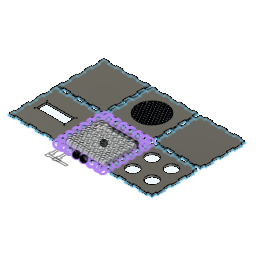
Alarm Clock v4 (Autodesk Fusion 360 design; units mm, degrees)
Autodesk Fusion 360 part; units mm, degrees
(part 1 of 3)
sketch "box (5)" plane through (0, 0, 0) normal (0, 0, 1) x (1, 0, 0)
  line L0 (0, 72.1875) -> (3, 72.1875)
  line L1 (0, 17.0625) -> (0, 3)
  line L2 (3, 108.9375) -> (3, 90.5625)
  line L3 (3, 35.4375) -> (3, 17.0625)
  line L4 (0, 108.9375) -> (3, 108.9375)
  line L5 (3, 72.1875) -> (3, 53.8125)
  line L6 (3, 53.8125) -> (0, 53.8125)
  line L7 (0, 35.4375) -> (3, 35.4375)
  line L8 (3, 17.0625) -> (0, 17.0625)
  line L9 (3, 90.5625) -> (0, 90.5625)
  line L10 (0, 123) -> (0, 108.9375)
  line L11 (0, 53.8125) -> (0, 35.4375)
  line L12 (117, 35.4375) -> (120, 35.4375)
  line L13 (120, 123) -> (105.9375, 123)
  line L14 (32.4375, 3) -> (50.8125, 3)
  line L15 (50.8125, 6) -> (69.1875, 6)
  line L16 (69.1875, 6) -> (69.1875, 3)
  line L17 (120, 108.9375) -> (120, 123)
  line L18 (87.5625, 3) -> (87.5625, 6)
  line L19 (120, 3) -> (120, 17.0625)
  line L20 (120, 53.8125) -> (117, 53.8125)
  line L21 (117, 53.8125) -> (117, 72.1875)
  line L22 (0, 90.5625) -> (0, 72.1875)
  line L23 (69.1875, 3) -> (87.5625, 3)
  line L24 (120, 90.5625) -> (117, 90.5625)
  line L25 (0, 3) -> (14.0625, 3)
  line L26 (87.5625, 123) -> (69.1875, 123)
  line L27 (50.8125, 3) -> (50.8125, 6)
  line L28 (87.5625, 120) -> (87.5625, 123)
  line L29 (87.5625, 6) -> (105.9375, 6)
  line L30 (105.9375, 6) -> (105.9375, 3)
  line L31 (120, 35.4375) -> (120, 53.8125)
  line L32 (120, 17.0625) -> (117, 17.0625)
  line L33 (120, 72.1875) -> (120, 90.5625)
  line L34 (105.9375, 120) -> (87.5625, 120)
  line L35 (32.4375, 6) -> (32.4375, 3)
  line L36 (14.0625, 3) -> (14.0625, 6)
  line L37 (117, 17.0625) -> (117, 35.4375)
  line L38 (117, 90.5625) -> (117, 108.9375)
  line L39 (105.9375, 123) -> (105.9375, 120)
  line L40 (14.0625, 6) -> (32.4375, 6)
  line L41 (105.9375, 3) -> (120, 3)
  line L42 (117, 72.1875) -> (120, 72.1875)
  line L43 (117, 108.9375) -> (120, 108.9375)
  line L44 (69.1875, 123) -> (69.1875, 120)
  line L45 (14.0625, 123) -> (0, 123)
  line L46 (14.0625, 120) -> (14.0625, 123)
  line L47 (32.4375, 123) -> (32.4375, 120)
  line L48 (32.4375, 120) -> (14.0625, 120)
  line L49 (50.8125, 123) -> (32.4375, 123)
  line L50 (50.8125, 120) -> (50.8125, 123)
  line L51 (69.1875, 120) -> (50.8125, 120)
  line L52 (210.5625, 123) -> (192.1875, 123)
  line L53 (173.8125, 3) -> (173.8125, 6)
  line L54 (240, 123) -> (228.9375, 123)
  line L55 (210.5625, 3) -> (210.5625, 6)
  line L56 (243, 35.4375) -> (240, 35.4375)
  line L57 (123, 90.5625) -> (126, 90.5625)
  line L58 (210.5625, 6) -> (228.9375, 6)
  line L59 (126, 3) -> (137.0625, 3)
  line L60 (192.1875, 123) -> (192.1875, 120)
  line L61 (123, 35.4375) -> (123, 17.0625)
  line L62 (123, 17.0625) -> (126, 17.0625)
  line L63 (126, 108.9375) -> (123, 108.9375)
  line L64 (126, 90.5625) -> (126, 72.1875)
  line L65 (240, 108.9375) -> (240, 123)
  line L66 (243, 72.1875) -> (240, 72.1875)
  line L67 (155.4375, 6) -> (155.4375, 3)
  line L68 (173.8125, 120) -> (173.8125, 123)
  line L69 (123, 72.1875) -> (123, 53.8125)
  line L70 (240, 3) -> (240, 17.0625)
  line L71 (126, 53.8125) -> (126, 35.4375)
  line L72 (126, 17.0625) -> (126, 3)
  line L73 (243, 17.0625) -> (243, 35.4375)
  line L74 (228.9375, 6) -> (228.9375, 3)
  line L75 (123, 108.9375) -> (123, 90.5625)
  line L76 (192.1875, 6) -> (192.1875, 3)
  line L77 (155.4375, 3) -> (173.8125, 3)
  line L78 (137.0625, 6) -> (155.4375, 6)
  line L79 (173.8125, 6) -> (192.1875, 6)
  line L80 (228.9375, 120) -> (210.5625, 120)
  line L81 (126, 123) -> (126, 108.9375)
  line L82 (137.0625, 3) -> (137.0625, 6)
  line L83 (126, 35.4375) -> (123, 35.4375)
  line L84 (126, 72.1875) -> (123, 72.1875)
  line L85 (123, 53.8125) -> (126, 53.8125)
  line L86 (240, 17.0625) -> (243, 17.0625)
  line L87 (240, 35.4375) -> (240, 53.8125)
  line L88 (243, 108.9375) -> (240, 108.9375)
  line L89 (173.8125, 123) -> (155.4375, 123)
  line L90 (240, 53.8125) -> (243, 53.8125)
  line L91 (192.1875, 120) -> (173.8125, 120)
  line L92 (243, 53.8125) -> (243, 72.1875)
  line L93 (240, 90.5625) -> (243, 90.5625)
  line L94 (240, 72.1875) -> (240, 90.5625)
  line L95 (137.0625, 123) -> (126, 123)
  line L96 (155.4375, 120) -> (137.0625, 120)
  line L97 (210.5625, 120) -> (210.5625, 123)
  line L98 (243, 90.5625) -> (243, 108.9375)
  line L99 (155.4375, 123) -> (155.4375, 120)
  line L100 (228.9375, 3) -> (240, 3)
  line L101 (137.0625, 120) -> (137.0625, 123)
  line L102 (228.9375, 123) -> (228.9375, 120)
  line L103 (192.1875, 3) -> (210.5625, 3)
  line L104 (249, 120) -> (249, 108.9375)
  line L105 (260.0625, 6) -> (260.0625, 3)
  line L106 (351.9375, 3) -> (351.9375, 6)
  line L107 (296.8125, 6) -> (296.8125, 3)
  line L108 (278.4375, 6) -> (296.8125, 6)
  line L109 (366, 72.1875) -> (363, 72.1875)
  line L110 (363, 108.9375) -> (363, 120)
  line L111 (333.5625, 6) -> (333.5625, 3)
  line L112 (249, 17.0625) -> (249, 6)
  line L113 (278.4375, 3) -> (278.4375, 6)
  line L114 (351.9375, 6) -> (363, 6)
  line L115 (333.5625, 120) -> (315.1875, 120)
  line L116 (366, 108.9375) -> (363, 108.9375)
  line L117 (246, 72.1875) -> (246, 53.8125)
  line L118 (351.9375, 120) -> (351.9375, 123)
  line L119 (246, 17.0625) -> (249, 17.0625)
  line L120 (315.1875, 120) -> (315.1875, 123)
  line L121 (296.8125, 123) -> (296.8125, 120)
  line L122 (260.0625, 120) -> (249, 120)
  line L123 (366, 90.5625) -> (366, 108.9375)
  line L124 (249, 90.5625) -> (249, 72.1875)
  line L125 (246, 108.9375) -> (246, 90.5625)
  line L126 (366, 35.4375) -> (363, 35.4375)
  line L127 (246, 90.5625) -> (249, 90.5625)
  line L128 (363, 35.4375) -> (363, 53.8125)
  line L129 (296.8125, 3) -> (315.1875, 3)
  line L130 (278.4375, 123) -> (260.0625, 123)
  line L131 (249, 6) -> (260.0625, 6)
  line L132 (315.1875, 6) -> (333.5625, 6)
  line L133 (246, 53.8125) -> (249, 53.8125)
  line L134 (260.0625, 3) -> (278.4375, 3)
  line L135 (363, 120) -> (351.9375, 120)
  line L136 (363, 6) -> (363, 17.0625)
  line L137 (333.5625, 123) -> (333.5625, 120)
  line L138 (249, 108.9375) -> (246, 108.9375)
  line L139 (363, 90.5625) -> (366, 90.5625)
  line L140 (315.1875, 123) -> (296.8125, 123)
  line L141 (363, 72.1875) -> (363, 90.5625)
  line L142 (366, 53.8125) -> (366, 72.1875)
  line L143 (315.1875, 3) -> (315.1875, 6)
  line L144 (296.8125, 120) -> (278.4375, 120)
  line L145 (249, 53.8125) -> (249, 35.4375)
  line L146 (260.0625, 123) -> (260.0625, 120)
  line L147 (278.4375, 120) -> (278.4375, 123)
  line L148 (249, 35.4375) -> (246, 35.4375)
  line L149 (246, 35.4375) -> (246, 17.0625)
  line L150 (249, 72.1875) -> (246, 72.1875)
  line L151 (333.5625, 3) -> (351.9375, 3)
  line L152 (351.9375, 123) -> (333.5625, 123)
  line L153 (363, 17.0625) -> (366, 17.0625)
  line L154 (363, 53.8125) -> (366, 53.8125)
  line L155 (366, 17.0625) -> (366, 35.4375)
  line L156 (3, 213.5625) -> (0, 213.5625)
  line L157 (0, 231.9375) -> (3, 231.9375)
  line L158 (3, 231.9375) -> (3, 213.5625)
  line L159 (0, 195.1875) -> (3, 195.1875)
  line L160 (32.4375, 243) -> (14.0625, 243)
  line L161 (14.0625, 129) -> (32.4375, 129)
  line L162 (0, 140.0625) -> (0, 126)
  line L163 (69.1875, 126) -> (87.5625, 126)
  line L164 (50.8125, 126) -> (50.8125, 129)
  line L165 (69.1875, 129) -> (69.1875, 126)
  line L166 (120, 176.8125) -> (117, 176.8125)
  line L167 (117, 140.0625) -> (117, 158.4375)
  line L168 (0, 176.8125) -> (0, 158.4375)
  line L169 (14.0625, 246) -> (0, 246)
  line L170 (87.5625, 126) -> (87.5625, 129)
  line L171 (3, 195.1875) -> (3, 176.8125)
  line L172 (50.8125, 243) -> (50.8125, 246)
  line L173 (0, 213.5625) -> (0, 195.1875)
  line L174 (69.1875, 243) -> (50.8125, 243)
  line L175 (120, 246) -> (105.9375, 246)
  line L176 (117, 231.9375) -> (120, 231.9375)
  line L177 (120, 158.4375) -> (120, 176.8125)
  line L178 (87.5625, 129) -> (105.9375, 129)
  line L179 (32.4375, 126) -> (50.8125, 126)
  line L180 (0, 126) -> (14.0625, 126)
  line L181 (32.4375, 129) -> (32.4375, 126)
  line L182 (105.9375, 246) -> (105.9375, 243)
  line L183 (105.9375, 243) -> (87.5625, 243)
  line L184 (120, 140.0625) -> (117, 140.0625)
  line L185 (87.5625, 243) -> (87.5625, 246)
  line L186 (87.5625, 246) -> (69.1875, 246)
  line L187 (3, 158.4375) -> (3, 140.0625)
  line L188 (120, 195.1875) -> (120, 213.5625)
  line L189 (117, 213.5625) -> (117, 231.9375)
  line L190 (117, 195.1875) -> (120, 195.1875)
  line L191 (69.1875, 246) -> (69.1875, 243)
  line L192 (32.4375, 246) -> (32.4375, 243)
  line L193 (0, 158.4375) -> (3, 158.4375)
  line L194 (50.8125, 129) -> (69.1875, 129)
  line L195 (14.0625, 126) -> (14.0625, 129)
  line L196 (120, 126) -> (120, 140.0625)
  line L197 (120, 213.5625) -> (117, 213.5625)
  line L198 (3, 140.0625) -> (0, 140.0625)
  line L199 (105.9375, 129) -> (105.9375, 126)
  line L200 (3, 176.8125) -> (0, 176.8125)
  line L201 (117, 176.8125) -> (117, 195.1875)
  line L202 (0, 246) -> (0, 231.9375)
  line L203 (14.0625, 243) -> (14.0625, 246)
  line L204 (50.8125, 246) -> (32.4375, 246)
  line L205 (120, 231.9375) -> (120, 246)
  line L206 (117, 158.4375) -> (120, 158.4375)
  line L207 (105.9375, 126) -> (120, 126)
  line L208 (126, 140.0625) -> (126, 126)
  line L209 (123, 140.0625) -> (126, 140.0625)
  line L210 (123, 158.4375) -> (123, 140.0625)
  line L211 (126, 158.4375) -> (123, 158.4375)
  line L212 (126, 195.1875) -> (123, 195.1875)
  line L213 (123, 213.5625) -> (126, 213.5625)
  line L214 (126, 231.9375) -> (123, 231.9375)
  line L215 (123, 176.8125) -> (126, 176.8125)
  line L216 (126, 176.8125) -> (126, 158.4375)
  line L217 (123, 195.1875) -> (123, 176.8125)
  line L218 (126, 213.5625) -> (126, 195.1875)
  line L219 (126, 246) -> (126, 231.9375)
  line L220 (137.0625, 126) -> (137.0625, 129)
  line L221 (173.8125, 126) -> (173.8125, 129)
  line L222 (192.1875, 129) -> (192.1875, 126)
  line L223 (137.0625, 129) -> (155.4375, 129)
  line L224 (155.4375, 126) -> (173.8125, 126)
  line L225 (123, 231.9375) -> (123, 213.5625)
  line L226 (240, 213.5625) -> (243, 213.5625)
  line L227 (240, 246) -> (228.9375, 246)
  line L228 (240, 158.4375) -> (240, 176.8125)
  line L229 (192.1875, 246) -> (192.1875, 243)
  line L230 (126, 126) -> (137.0625, 126)
  line L231 (243, 195.1875) -> (240, 195.1875)
  line L232 (228.9375, 129) -> (228.9375, 126)
  line L233 (243, 176.8125) -> (243, 195.1875)
  line L234 (137.0625, 246) -> (126, 246)
  line L235 (228.9375, 126) -> (240, 126)
  line L236 (210.5625, 126) -> (210.5625, 129)
  line L237 (240, 195.1875) -> (240, 213.5625)
  line L238 (228.9375, 246) -> (228.9375, 243)
  line L239 (243, 213.5625) -> (243, 231.9375)
  line L240 (155.4375, 246) -> (155.4375, 243)
  line L241 (240, 231.9375) -> (240, 246)
  line L242 (228.9375, 243) -> (210.5625, 243)
  line L243 (240, 126) -> (240, 140.0625)
  line L244 (243, 158.4375) -> (240, 158.4375)
  line L245 (243, 231.9375) -> (240, 231.9375)
  line L246 (155.4375, 243) -> (137.0625, 243)
  line L247 (210.5625, 129) -> (228.9375, 129)
  line L248 (240, 140.0625) -> (243, 140.0625)
  line L249 (137.0625, 243) -> (137.0625, 246)
  line L250 (192.1875, 243) -> (173.8125, 243)
  line L251 (155.4375, 129) -> (155.4375, 126)
  line L252 (192.1875, 126) -> (210.5625, 126)
  line L253 (173.8125, 129) -> (192.1875, 129)
  line L254 (243, 140.0625) -> (243, 158.4375)
  line L255 (210.5625, 246) -> (192.1875, 246)
  line L256 (210.5625, 243) -> (210.5625, 246)
  line L257 (240, 176.8125) -> (243, 176.8125)
  line L258 (173.8125, 246) -> (155.4375, 246)
  line L259 (173.8125, 243) -> (173.8125, 246)
  line L260 (296.8125, 129) -> (296.8125, 126)
  line L261 (260.0625, 126) -> (278.4375, 126)
  line L262 (278.4375, 126) -> (278.4375, 129)
  line L263 (249, 176.8125) -> (249, 158.4375)
  line L264 (249, 195.1875) -> (246, 195.1875)
  line L265 (296.8125, 126) -> (315.1875, 126)
  line L266 (249, 140.0625) -> (249, 129)
  line L267 (246, 231.9375) -> (246, 213.5625)
  line L268 (249, 129) -> (260.0625, 129)
  line L269 (246, 140.0625) -> (249, 140.0625)
  line L270 (246, 195.1875) -> (246, 176.8125)
  line L271 (278.4375, 129) -> (296.8125, 129)
  line L272 (315.1875, 126) -> (315.1875, 129)
  line L273 (260.0625, 129) -> (260.0625, 126)
  line L274 (315.1875, 129) -> (333.5625, 129)
  line L275 (333.5625, 129) -> (333.5625, 126)
  line L276 (246, 158.4375) -> (246, 140.0625)
  line L277 (249, 213.5625) -> (249, 195.1875)
  line L278 (351.9375, 246) -> (333.5625, 246)
  line L279 (249, 231.9375) -> (246, 231.9375)
  line L280 (333.5625, 126) -> (351.9375, 126)
  line L281 (249, 243) -> (249, 231.9375)
  line L282 (246, 213.5625) -> (249, 213.5625)
  line L283 (351.9375, 126) -> (351.9375, 129)
  line L284 (246, 176.8125) -> (249, 176.8125)
  line L285 (249, 158.4375) -> (246, 158.4375)
  line L286 (363, 176.8125) -> (366, 176.8125)
  line L287 (296.8125, 243) -> (278.4375, 243)
  line L288 (351.9375, 129) -> (363, 129)
  line L289 (278.4375, 246) -> (260.0625, 246)
  line L290 (296.8125, 246) -> (296.8125, 243)
  line L291 (363, 243) -> (351.9375, 243)
  line L292 (278.4375, 243) -> (278.4375, 246)
  line L293 (315.1875, 243) -> (315.1875, 246)
  line L294 (366, 140.0625) -> (366, 158.4375)
  line L295 (363, 158.4375) -> (363, 176.8125)
  line L296 (363, 231.9375) -> (363, 243)
  line L297 (366, 158.4375) -> (363, 158.4375)
  line L298 (363, 213.5625) -> (366, 213.5625)
  line L299 (366, 176.8125) -> (366, 195.1875)
  line L300 (363, 195.1875) -> (363, 213.5625)
  line L301 (315.1875, 246) -> (296.8125, 246)
  line L302 (351.9375, 243) -> (351.9375, 246)
  line L303 (363, 129) -> (363, 140.0625)
  line L304 (366, 231.9375) -> (363, 231.9375)
  line L305 (366, 195.1875) -> (363, 195.1875)
  line L306 (333.5625, 246) -> (333.5625, 243)
  line L307 (260.0625, 246) -> (260.0625, 243)
  line L308 (260.0625, 243) -> (249, 243)
  line L309 (363, 140.0625) -> (366, 140.0625)
  line L310 (366, 213.5625) -> (366, 231.9375)
  line L311 (333.5625, 243) -> (315.1875, 243)
sketch "Sketch2" plane through (0, 0, 0) normal (0, 0, 1) x (1, 0, 0)
  line L0 (246, 108.9375) -> (246, 90.5625)
  line L1 (249, 108.9375) -> (246, 108.9375)
  line L2 (249, 120) -> (249, 108.9375)
  line L3 (260.0625, 120) -> (249, 120)
  line L4 (278.4375, 123) -> (260.0625, 123)
  line L5 (260.0625, 123) -> (260.0625, 120)
  line L6 (278.4375, 120) -> (278.4375, 123)
  line L7 (351.9375, 123) -> (333.5625, 123)
  line L8 (363, 120) -> (351.9375, 120)
  line L9 (366, 90.5625) -> (366, 108.9375)
  line L10 (363, 108.9375) -> (363, 120)
  line L11 (366, 108.9375) -> (363, 108.9375)
  line L12 (351.9375, 120) -> (351.9375, 123)
  line L13 (249, 17.0625) -> (249, 6)
  line L14 (246, 17.0625) -> (249, 17.0625)
  line L15 (246, 35.4375) -> (246, 17.0625)
  line L16 (249, 6) -> (260.0625, 6)
  line L17 (260.0625, 6) -> (260.0625, 3)
  line L18 (260.0625, 3) -> (278.4375, 3)
  line L19 (333.5625, 3) -> (351.9375, 3)
  line L20 (351.9375, 3) -> (351.9375, 6)
  line L21 (351.9375, 6) -> (363, 6)
  line L22 (363, 6) -> (363, 17.0625)
  line L23 (363, 17.0625) -> (366, 17.0625)
  line L24 (366, 17.0625) -> (366, 35.4375)
  line L25 (260.0625, 123) -> (240, 123)
  line L26 (246, 108.9375) -> (246, 123)
  line L27 (351.9375, 123) -> (370, 123)
  line L28 (366, 108.9375) -> (366, 123)
  line L29 (246, 17.0625) -> (246, 0)
  line L30 (260.0625, 3) -> (246, 3)
  line L31 (351.9375, 3) -> (370, 3)
  line L32 (366, 17.0625) -> (366, 3)
  circle A0 centre (281.3553, 38.3553) radius 15
  line L33 (281.3553, 38.3553) -> (246, 3) construction
  circle A1 centre (330.6447, 38.3553) radius 15
  line L34 (330.6447, 38.3553) -> (366, 3) construction
  circle A2 centre (330.6447, 87.6447) radius 15
  line L35 (366, 123) -> (330.6447, 87.6447) construction
  circle A3 centre (281.3553, 87.6447) radius 15
  line L36 (246, 123) -> (281.3553, 87.6447) construction
  line L37 (246, 90.5625) -> (249, 90.5625)
  line L38 (249, 90.5625) -> (249, 72.1875)
  line L39 (249, 72.1875) -> (246, 72.1875)
  line L40 (246, 72.1875) -> (246, 53.8125)
  line L41 (246, 53.8125) -> (249, 53.8125)
  line L42 (249, 53.8125) -> (249, 35.4375)
  line L43 (249, 35.4375) -> (246, 35.4375)
  line L44 (296.8125, 120) -> (278.4375, 120)
  line L45 (315.1875, 123) -> (296.8125, 123)
  line L46 (296.8125, 123) -> (296.8125, 120)
  line L47 (315.1875, 120) -> (315.1875, 123)
  line L48 (333.5625, 120) -> (315.1875, 120)
  line L49 (333.5625, 123) -> (333.5625, 120)
  line L50 (363, 90.5625) -> (366, 90.5625)
  line L51 (363, 72.1875) -> (363, 90.5625)
  line L52 (366, 72.1875) -> (363, 72.1875)
  line L53 (366, 53.8125) -> (366, 72.1875)
  line L54 (363, 35.4375) -> (363, 53.8125)
  line L55 (363, 53.8125) -> (366, 53.8125)
  line L56 (366, 35.4375) -> (363, 35.4375)
  line L57 (333.5625, 6) -> (333.5625, 3)
  line L58 (315.1875, 6) -> (333.5625, 6)
  line L59 (315.1875, 3) -> (315.1875, 6)
  line L60 (296.8125, 3) -> (315.1875, 3)
  line L61 (296.8125, 6) -> (296.8125, 3)
  line L62 (278.4375, 6) -> (296.8125, 6)
  line L63 (278.4375, 3) -> (278.4375, 6)
  point P0 (249, 120)
  point P1 (249, 108.9375)
  point P2 (246, 108.9375)
  point P3 (246, 90.5625)
  point P4 (249, 90.5625)
  point P5 (249, 72.1875)
  point P6 (246, 72.1875)
  point P7 (246, 53.8125)
  point P8 (249, 53.8125)
  point P9 (249, 35.4375)
  point P10 (246, 35.4375)
  point P11 (246, 17.0625)
  point P12 (249, 17.0625)
  point P13 (249, 6)
  point P14 (260.0625, 6)
  point P15 (260.0625, 3)
  point P16 (278.4375, 3)
  point P17 (278.4375, 6)
  point P18 (296.8125, 6)
  point P19 (296.8125, 3)
  point P20 (315.1875, 3)
  point P21 (315.1875, 6)
  point P22 (333.5625, 6)
  point P23 (333.5625, 3)
  point P24 (351.9375, 3)
  point P25 (351.9375, 6)
  point P26 (363, 6)
  point P27 (363, 17.0625)
  point P28 (366, 17.0625)
  point P29 (366, 35.4375)
  point P30 (363, 35.4375)
  point P31 (363, 53.8125)
  point P32 (366, 53.8125)
  point P33 (366, 72.1875)
  point P34 (363, 72.1875)
  point P35 (363, 90.5625)
  point P36 (366, 90.5625)
  point P37 (366, 108.9375)
  point P38 (363, 108.9375)
  point P39 (363, 120)
  point P40 (351.9375, 120)
  point P41 (351.9375, 123)
  point P42 (333.5625, 123)
  point P43 (333.5625, 120)
  point P44 (315.1875, 120)
  point P45 (315.1875, 123)
  point P46 (296.8125, 123)
  point P47 (296.8125, 120)
  point P48 (278.4375, 120)
  point P49 (278.4375, 123)
  point P50 (260.0625, 123)
  point P51 (260.0625, 120)
  dimension "d1" = 30
  dimension "d2" = 50
  dimension "d3" = 45
  dimension "d4" = 30
  dimension "d5" = 50
  dimension "d6" = 45
  dimension "d7" = 30
  dimension "d8" = 50
  dimension "d9" = 45
  dimension "d10" = 30
  dimension "d11" = 50
  dimension "d12" = 45
  constraint coincident P50 L4.end
  constraint perpendicular L5 L25
  constraint coincident P2 L0.start
  constraint coincident L25 L26.end
  constraint perpendicular L25 L26
  constraint coincident P41 L7.start
  constraint perpendicular L12 L27
  constraint coincident P37 L9.end
  constraint coincident L27 L28.end
  constraint perpendicular L27 L28
  constraint coincident P11 L14.start
  constraint perpendicular L14 L29
  constraint coincident P15 L17.end
  constraint coincident L29 L30.end
  constraint perpendicular L29 L30
  constraint coincident P24 L19.end
  constraint perpendicular L20 L31
  constraint coincident P28 L23.end
  constraint coincident L31 L32.end
  constraint perpendicular L31 L32
  constraint coincident A0.centre L33.start
  constraint coincident A1.centre L34.start
  constraint coincident A2.centre L35.end
  constraint coincident A3.centre L36.end
  measures "d1" diameter of A0
  measures "d2" distance of L30.end A0.centre
  measures "d3" angle of L30 L33
  measures "d4" diameter of A1
  measures "d5" distance of L32.end A1.centre
  measures "d6" angle of L31 L34
  measures "d7" diameter of A2
  measures "d8" distance of L28.end A2.centre
  measures "d9" angle of L27 L35
  measures "d10" diameter of A3
  measures "d11" distance of L26.end A3.centre
  measures "d12" angle of L25 L36
extrude "Extrude1" add sketch "Sketch2" along normal blind 5.2 contours L0 L1 L2 L3 L4 L5 L6 L7 L8 L9 L10 L11 L12 L13 L14 L15 L16 L17 L18 L19 L20 L21 L22 L23 L24 L37 L38 L39 L40 L41 L42 L43 L44 L45 L46 L47 L48 L49 L50 L51 L52 L53 L54 L55 L56 L57 L58 L59 L60 L61 L62 L63 makes body 1
sketch "Sketch3" plane through (0, 0, 0) normal (0, 0, 1) x (1, 0, 0)
  line L0 (0, 123) -> (0, 108.9375)
  line L1 (14.0625, 123) -> (0, 123)
  line L2 (14.0625, 120) -> (14.0625, 123)
  line L3 (32.4375, 120) -> (14.0625, 120)
  line L4 (32.4375, 123) -> (32.4375, 120)
  line L5 (50.8125, 123) -> (32.4375, 123)
  line L6 (50.8125, 120) -> (50.8125, 123)
  line L7 (69.1875, 120) -> (50.8125, 120)
  line L8 (69.1875, 123) -> (69.1875, 120)
  line L9 (87.5625, 123) -> (69.1875, 123)
  line L10 (87.5625, 120) -> (87.5625, 123)
  line L11 (105.9375, 120) -> (87.5625, 120)
  line L12 (105.9375, 123) -> (105.9375, 120)
  line L13 (120, 123) -> (105.9375, 123)
  line L14 (120, 108.9375) -> (120, 123)
  line L15 (117, 108.9375) -> (120, 108.9375)
  line L16 (117, 90.5625) -> (117, 108.9375)
  line L17 (120, 90.5625) -> (117, 90.5625)
  line L18 (120, 72.1875) -> (120, 90.5625)
  line L19 (117, 53.8125) -> (117, 72.1875)
  line L20 (117, 72.1875) -> (120, 72.1875)
  line L21 (120, 53.8125) -> (117, 53.8125)
  line L22 (120, 35.4375) -> (120, 53.8125)
  line L23 (117, 35.4375) -> (120, 35.4375)
  line L24 (117, 17.0625) -> (117, 35.4375)
  line L25 (120, 17.0625) -> (117, 17.0625)
  line L26 (105.9375, 6) -> (105.9375, 3)
  line L27 (120, 3) -> (120, 17.0625)
  line L28 (105.9375, 3) -> (120, 3)
  line L29 (87.5625, 6) -> (105.9375, 6)
  line L30 (87.5625, 3) -> (87.5625, 6)
  line L31 (69.1875, 3) -> (87.5625, 3)
  line L32 (69.1875, 6) -> (69.1875, 3)
  line L33 (50.8125, 6) -> (69.1875, 6)
  line L34 (50.8125, 3) -> (50.8125, 6)
  line L35 (32.4375, 6) -> (32.4375, 3)
  line L36 (32.4375, 3) -> (50.8125, 3)
  line L37 (14.0625, 6) -> (32.4375, 6)
  line L38 (14.0625, 3) -> (14.0625, 6)
  line L39 (0, 3) -> (14.0625, 3)
  line L40 (0, 17.0625) -> (0, 3)
  line L41 (3, 17.0625) -> (0, 17.0625)
  line L42 (3, 35.4375) -> (3, 17.0625)
  line L43 (0, 35.4375) -> (3, 35.4375)
  line L44 (0, 53.8125) -> (0, 35.4375)
  line L45 (3, 53.8125) -> (0, 53.8125)
  line L46 (0, 108.9375) -> (3, 108.9375)
  line L47 (3, 108.9375) -> (3, 90.5625)
  line L48 (3, 90.5625) -> (0, 90.5625)
  line L49 (0, 90.5625) -> (0, 72.1875)
  line L50 (0, 72.1875) -> (3, 72.1875)
  line L51 (3, 72.1875) -> (3, 53.8125)
  line L52 (0, 3) -> (120, 3) construction
  line L53 (0, 3) -> (0, 123) construction
  line L54 (0, 63) -> (20, 63) construction
  line L55 (120, 123) -> (120, 3) construction
  line L56 (120, 63) -> (100, 63) construction
  line L57 (100, 63) -> (100, 81) construction
  line L58 (100, 63) -> (100, 45) construction
  line L59 (20, 63) -> (20, 81) construction
  line L60 (20, 63) -> (20, 45) construction
  line L61 (20, 81) -> (100, 81) construction
  line L62 (20, 45) -> (100, 45) construction
  line L63 (20, 81) -> (100, 81)
  line L64 (100, 81) -> (100, 45)
  line L65 (100, 45) -> (20, 45)
  line L66 (20, 45) -> (20, 81)
  line L67 (20, 63) -> (24.4, 63) construction
  line L68 (100, 63) -> (95.6, 63) construction
  line L69 (60, 45) -> (60, 49.8) construction
  line L70 (60, 81) -> (60, 74.5) construction
  line L71 (24.4, 63) -> (24.4, 50.5) construction
  line L72 (24.4, 63) -> (24.4, 75.5) construction
  line L73 (95.6, 63) -> (95.6, 75.5) construction
  line L74 (95.6, 63) -> (95.6, 50.5) construction
  line L75 (24.4, 50.5) -> (95.6, 50.5)
  line L76 (24.4, 75.5) -> (95.6, 75.5)
  line L77 (95.6, 50.5) -> (95.6, 75.5)
  line L78 (24.4, 50.5) -> (24.4, 75.5)
  line L79 (100, 81) -> (99, 81) construction
  line L80 (99, 81) -> (99, 80) construction
  circle A0 centre (97.5, 78.5) radius 1.5
  line L81 (99, 80) -> (99, 45) construction
  line L82 (20, 81) -> (21, 81) construction
  line L83 (21, 81) -> (21, 45) construction
  line L84 (20, 81) -> (20, 80) construction
  line L85 (20, 80) -> (100, 80) construction
  line L86 (20, 45) -> (20, 46) construction
  line L87 (20, 46) -> (100, 46) construction
  line L88 (100, 45) -> (100, 46) construction
  line L89 (97.5, 78.5) -> (99, 78.5) construction
  line L90 (97.5, 78.5) -> (97.5, 80) construction
  line L91 (99, 80) -> (97.5, 80) construction
  line L92 (99, 80) -> (99, 78.5) construction
  line L93 (99, 46) -> (99, 47.5) construction
  circle A1 centre (97.5, 47.5) radius 1.5
  line L94 (97.5, 47.5) -> (97.5, 46) construction
  line L95 (97.5, 47.5) -> (99, 47.5) construction
  line L96 (21, 46) -> (21, 47.5) construction
  circle A2 centre (22.5, 47.5) radius 1.5
  line L97 (22.5, 47.5) -> (22.5, 46) construction
  line L98 (22.5, 47.5) -> (21, 47.5) construction
  line L99 (21, 80) -> (22.5, 80) construction
  circle A3 centre (22.5, 78.5) radius 1.5
  line L100 (22.5, 78.5) -> (22.5, 80) construction
  dimension "d15" = 20
  dimension "d16" = 20
  dimension "d17" = 18
  dimension "d18" = 18
  dimension "d19" = 18
  dimension "d20" = 18
  dimension "d21" = 4.4
  dimension "d22" = 4.4
  dimension "d23" = 4.8
  dimension "d24" = 6.5
  dimension "d25" = 12.5
  dimension "d26" = 12.5
  dimension "d27" = 12.5
  dimension "d28" = 12.5
  dimension "d29" = 3
  dimension "d30" = 1.5
  dimension "d31" = 1.5
  dimension "d32" = 1.5
  dimension "d33" = 3
  dimension "d34" = 1.5
  dimension "d35" = 3
  dimension "d36" = 1.5
  dimension "d37" = 3
  dimension "d38" = 2.5
  dimension "d39" = 2.5
  dimension "d40" = 2.5
  dimension "d41" = 2.5
  dimension "d42" = 2.5
  dimension "d43" = 2.5
  dimension "d44" = 2.5
  dimension "d45" = 2.5
  constraint coincident L39.start L40.end
  constraint coincident L27.start L28.end
  constraint coincident L0.start L1.end
  constraint midpoint L53 L54.start
  constraint perpendicular L53 L54
  constraint coincident L13.start L14.end
  constraint midpoint L55 L56.start
  constraint perpendicular L19 L56
  constraint perpendicular L56 L57
  constraint perpendicular L56 L58
  constraint perpendicular L54 L59
  constraint perpendicular L54 L60
  constraint perpendicular L59 L67
  constraint perpendicular L64 L68
  constraint midpoint L62 L69.start
  constraint perpendicular L65 L69
  constraint midpoint L61 L70.start
  constraint perpendicular L61 L70
  constraint perpendicular L67 L71
  constraint perpendicular L67 L72
  constraint perpendicular L68 L73
  constraint perpendicular L68 L74
  constraint coincident L63 L79.end
  constraint perpendicular L57 L79
  constraint perpendicular L79 L80
  constraint coincident L65 L81.end
  constraint perpendicular L65 L81
  constraint coincident L63 L82.end
  constraint perpendicular L66 L82
  constraint coincident L65 L83.end
  constraint perpendicular L65 L83
  constraint coincident L59 L84.end
  constraint coincident L57 L85.end
  constraint coincident L66 L86.end
  constraint perpendicular L65 L86
  constraint coincident L64 L87.end
  constraint coincident A0.centre L89.start
  constraint coincident A0 L89.end
  constraint horizontal L89
  constraint coincident A0 L90.end
  constraint perpendicular L89 L90
  constraint perpendicular L80 L91
  constraint perpendicular L85 L92
  constraint coincident L81 L93.start
  constraint coincident L87 L93.start
  constraint perpendicular L87 L93
  constraint coincident A1.centre L94.start
  constraint coincident A1 L94.end
  constraint vertical L94
  constraint coincident A1 L93.end
  constraint perpendicular L94 L95
  constraint coincident L83 L96.start
  constraint coincident L87 L96.start
  constraint perpendicular L87 L96
  constraint coincident A2.centre L97.start
  constraint coincident A2 L97.end
  constraint vertical L97
  constraint coincident A2 L96.end
  constraint perpendicular L97 L98
  constraint coincident L83 L99.start
  constraint coincident L85 L99.start
  constraint perpendicular L83 L99
  constraint coincident A3.centre L100.start
  constraint coincident A3 L99.end
  constraint perpendicular L85 L100
  measures "d15" distance of L54.start L54.end
  measures "d16" distance of L56.start L56.end
  measures "d17" distance of L56.end L57.end
  measures "d18" distance of L56.end L58.end
  measures "d19" distance of L54.end L59.end
  measures "d20" distance of L54.end L60.end
  measures "d21" distance of L54.end L67.end
  measures "d22" distance of L56.end L68.end
  measures "d23" distance of L69.start L69.end
  measures "d24" distance of L70.start L70.end
  measures "d25" distance of L67.end L71.end
  measures "d26" distance of L67.end L72.end
  measures "d27" distance of L68.end L73.end
  measures "d28" distance of L68.end L74.end
  measures "d29" diameter of A0
  measures "d30" distance of L80.end L90.end
  measures "d31" distance of L80.end L89.end
  measures "d32" distance of L93.start L93.end
  measures "d33" diameter of A1
  measures "d34" distance of L96.start L96.end
  measures "d35" diameter of A2
  measures "d36" distance of L99.start L99.end
  measures "d37" diameter of A3
  measures "d38" distance of L61 A3.centre
  measures "d39" distance of L66 A3.centre
  measures "d40" distance of L63 A0.centre
  measures "d41" distance of L57 A0.centre
  measures "d42" distance of L58 A1.centre
  measures "d43" distance of L65 A1.centre
  measures "d44" distance of L62 A2.centre
  measures "d45" distance of L66 A2.centre
extrude "Extrude2" add sketch "Sketch3" along normal blind 5.2 separate body contours L0 L1 L2 L3 L4 L5 L6 L7 L8 L9 L10 L11 L12 L13 L14 L15 L16 L17 L18 L19 L20 L21 L22 L23 L24 L25 L26 L27 L28 L29 L30 L31 L32 L33 L34 L35 L36 L37 L38 L39 L40 L41 L42 L43 L44 L45 L46 L47 L48 L49 L50 L51 makes body 2
extrude "Extrude3" add sketch "Sketch3" along normal blind 5.2 contours L63 L64 L65 L66 bodies 2
extrude "Extrude4" add sketch "box (5)" along normal blind 5.2 separate body contours L156 L157 L158 L159 L160 L161 L162 L163 L164 L165 L166 L167 L168 L169 L170 L171 L172 L173 L174 L175 L176 L177 L178 L179 L180 L181 L182 L183 L184 L185 L186 L187 L188 L189 L190 L191 L192 L193 L194 L195 L196 L197 L198 L199 L200 L201 L202 L203 L204 L205 L206 L207 | L260 L261 L262 L263 L264 L265 L266 L267 L268 L269 L270 L271 L272 L273 L274 L275 L276 L277 L278 L279 L280 L281 L282 L283 L284 L285 L286 L287 L288 L289 L290 L291 L292 L293 L294 L295 L296 L297 L298 L299 L300 L301 L302 L303 L304 L305 L306 L307 L308 L309 L310 L311 makes body 3 at (293.125, 189.0625, 0) makes body 4 at (79, 189.0625, 0)
sketch "Sketch4" plane through (0, 0, 0) normal (0, 0, 1) x (1, 0, 0)
  line L0 (123, 53.8125) -> (126, 53.8125)
  line L1 (126, 53.8125) -> (126, 35.4375)
  line L2 (126, 35.4375) -> (123, 35.4375)
  line L3 (123, 35.4375) -> (123, 17.0625)
  line L4 (123, 17.0625) -> (126, 17.0625)
  line L5 (126, 17.0625) -> (126, 3)
  line L6 (126, 3) -> (137.0625, 3)
  line L7 (137.0625, 3) -> (137.0625, 6)
  line L8 (137.0625, 6) -> (155.4375, 6)
  line L9 (155.4375, 6) -> (155.4375, 3)
  line L10 (155.4375, 3) -> (173.8125, 3)
  line L11 (173.8125, 3) -> (173.8125, 6)
  line L12 (173.8125, 6) -> (192.1875, 6)
  line L13 (192.1875, 6) -> (192.1875, 3)
  line L14 (210.5625, 3) -> (210.5625, 6)
  line L15 (192.1875, 3) -> (210.5625, 3)
  line L16 (137.0625, 123) -> (126, 123)
  line L17 (126, 123) -> (126, 108.9375)
  line L18 (126, 108.9375) -> (123, 108.9375)
  line L19 (123, 108.9375) -> (123, 90.5625)
  line L20 (123, 90.5625) -> (126, 90.5625)
  line L21 (126, 90.5625) -> (126, 72.1875)
  line L22 (126, 72.1875) -> (123, 72.1875)
  line L23 (123, 72.1875) -> (123, 53.8125)
  line L24 (210.5625, 6) -> (228.9375, 6)
  line L25 (228.9375, 6) -> (228.9375, 3)
  line L26 (228.9375, 3) -> (240, 3)
  line L27 (240, 3) -> (240, 17.0625)
  line L28 (240, 17.0625) -> (243, 17.0625)
  line L29 (243, 17.0625) -> (243, 35.4375)
  line L30 (243, 35.4375) -> (240, 35.4375)
  line L31 (240, 35.4375) -> (240, 53.8125)
  line L32 (240, 53.8125) -> (243, 53.8125)
  line L33 (243, 53.8125) -> (243, 72.1875)
  line L34 (243, 72.1875) -> (240, 72.1875)
  line L35 (240, 72.1875) -> (240, 90.5625)
  line L36 (240, 90.5625) -> (243, 90.5625)
  line L37 (243, 90.5625) -> (243, 108.9375)
  line L38 (155.4375, 120) -> (137.0625, 120)
  line L39 (137.0625, 120) -> (137.0625, 123)
  line L40 (155.4375, 123) -> (155.4375, 120)
  line L41 (173.8125, 123) -> (155.4375, 123)
  line L42 (173.8125, 120) -> (173.8125, 123)
  line L43 (192.1875, 120) -> (173.8125, 120)
  line L44 (192.1875, 123) -> (192.1875, 120)
  line L45 (210.5625, 123) -> (192.1875, 123)
  line L46 (210.5625, 120) -> (210.5625, 123)
  line L47 (228.9375, 120) -> (210.5625, 120)
  line L48 (228.9375, 123) -> (228.9375, 120)
  line L49 (240, 123) -> (228.9375, 123)
  line L50 (240, 108.9375) -> (240, 123)
  line L51 (243, 108.9375) -> (240, 108.9375)
  circle A0 centre (183, 63) radius 37.5
  line L52 (173.8125, 3) -> (192.1875, 3) construction
  line L53 (180.0127, 61.2461) -> (183.0252, 59.536)
  line L54 (183.0252, 59.536) -> (186.0125, 61.2898)
  line L55 (186.0125, 61.2898) -> (185.9873, 64.7539)
  line L56 (185.9873, 64.7539) -> (182.9748, 66.464)
  line L57 (182.9748, 66.464) -> (179.9875, 64.7102)
  line L58 (179.9875, 64.7102) -> (180.0127, 61.2461)
  line L59 (178.9875, 64.7005) -> (175.975, 66.4106)
  line L60 (175.975, 66.4106) -> (172.9877, 64.6567)
  line L61 (172.9877, 64.6567) -> (173.0129, 61.1927)
  line L62 (173.0129, 61.1927) -> (176.0254, 59.4826)
  line L63 (176.0254, 59.4826) -> (179.0127, 61.2364)
  line L64 (179.0127, 61.2364) -> (178.9875, 64.7005)
  line L65 (179.5211, 60.3753) -> (176.5338, 58.6214)
  line L66 (176.5338, 58.6214) -> (176.559, 55.1574)
  line L67 (176.559, 55.1574) -> (179.5716, 53.4473)
  line L68 (179.5716, 53.4473) -> (182.5589, 55.2011)
  line L69 (182.5589, 55.2011) -> (182.5337, 58.6652)
  line L70 (182.5337, 58.6652) -> (179.5211, 60.3753)
  line L71 (186.5209, 60.4287) -> (183.5336, 58.6749)
  line L72 (183.5336, 58.6749) -> (183.5588, 55.2108)
  line L73 (183.5588, 55.2108) -> (186.5714, 53.5007)
  line L74 (186.5714, 53.5007) -> (189.5587, 55.2545)
  line L75 (189.5587, 55.2545) -> (189.5335, 58.7186)
  line L76 (189.5335, 58.7186) -> (186.5209, 60.4287)
  line L77 (183, 63) -> (220.499, 63.2732)
  line L78 (140.5589, 19.2011) -> (140.5337, 22.6652)
  line L79 (143.9873, 28.7539) -> (140.9748, 30.464)
  line L80 (134.5338, 22.6214) -> (134.559, 19.1574)
  line L81 (131.0129, 25.1927) -> (134.0254, 23.4826)
  line L82 (140.9748, 30.464) -> (137.9875, 28.7102)
  line L83 (130.9877, 28.6567) -> (131.0129, 25.1927)
  line L84 (144.5714, 17.5007) -> (147.5587, 19.2545)
  line L85 (141.5336, 22.6749) -> (141.5588, 19.2108)
  line L86 (144.5209, 24.4287) -> (141.5336, 22.6749)
  line L87 (136.9875, 28.7005) -> (133.975, 30.4106)
  line L88 (137.5716, 17.4473) -> (140.5589, 19.2011)
  line L89 (140.5337, 22.6652) -> (137.5211, 24.3753)
  line L90 (137.9875, 28.7102) -> (138.0127, 25.2461)
  line L91 (134.0254, 23.4826) -> (137.0127, 25.2364)
  line L92 (141.5588, 19.2108) -> (144.5714, 17.5007)
  line L93 (137.5211, 24.3753) -> (134.5338, 22.6214)
  line L94 (138.0127, 25.2461) -> (141.0252, 23.536)
  line L95 (141.0252, 23.536) -> (144.0125, 25.2898)
  line L96 (137.0127, 25.2364) -> (136.9875, 28.7005)
  line L97 (133.975, 30.4106) -> (130.9877, 28.6567)
  line L98 (134.559, 19.1574) -> (137.5716, 17.4473)
  line L99 (144.0125, 25.2898) -> (143.9873, 28.7539)
  line L100 (147.5587, 19.2545) -> (147.5335, 22.7186)
  line L101 (147.5335, 22.7186) -> (144.5209, 24.4287)
  line L102 (154.5589, 19.2011) -> (154.5337, 22.6652)
  line L103 (157.9873, 28.7539) -> (154.9748, 30.464)
  line L104 (148.5338, 22.6214) -> (148.559, 19.1574)
  line L105 (145.0129, 25.1927) -> (148.0254, 23.4826)
  line L106 (154.9748, 30.464) -> (151.9875, 28.7102)
  line L107 (144.9877, 28.6567) -> (145.0129, 25.1927)
  line L108 (158.5714, 17.5007) -> (161.5587, 19.2545)
  line L109 (155.5336, 22.6749) -> (155.5588, 19.2108)
  line L110 (158.5209, 24.4287) -> (155.5336, 22.6749)
  line L111 (150.9875, 28.7005) -> (147.975, 30.4106)
  line L112 (151.5716, 17.4473) -> (154.5589, 19.2011)
  line L113 (154.5337, 22.6652) -> (151.5211, 24.3753)
  line L114 (151.9875, 28.7102) -> (152.0127, 25.2461)
  line L115 (148.0254, 23.4826) -> (151.0127, 25.2364)
  line L116 (155.5588, 19.2108) -> (158.5714, 17.5007)
  line L117 (151.5211, 24.3753) -> (148.5338, 22.6214)
  line L118 (152.0127, 25.2461) -> (155.0252, 23.536)
  line L119 (155.0252, 23.536) -> (158.0125, 25.2898)
  line L120 (151.0127, 25.2364) -> (150.9875, 28.7005)
  line L121 (147.975, 30.4106) -> (144.9877, 28.6567)
  line L122 (148.559, 19.1574) -> (151.5716, 17.4473)
  line L123 (158.0125, 25.2898) -> (157.9873, 28.7539)
  line L124 (161.5587, 19.2545) -> (161.5335, 22.7186)
  line L125 (161.5335, 22.7186) -> (158.5209, 24.4287)
  line L126 (168.5589, 19.2011) -> (168.5337, 22.6652)
  line L127 (171.9873, 28.7539) -> (168.9748, 30.464)
  line L128 (162.5338, 22.6214) -> (162.559, 19.1574)
  line L129 (159.0129, 25.1927) -> (162.0254, 23.4826)
  line L130 (168.9748, 30.464) -> (165.9875, 28.7102)
  line L131 (158.9877, 28.6567) -> (159.0129, 25.1927)
  line L132 (172.5714, 17.5007) -> (175.5587, 19.2545)
  line L133 (169.5336, 22.6749) -> (169.5588, 19.2108)
  line L134 (172.5209, 24.4287) -> (169.5336, 22.6749)
  line L135 (164.9875, 28.7005) -> (161.975, 30.4106)
  line L136 (165.5716, 17.4473) -> (168.5589, 19.2011)
  line L137 (168.5337, 22.6652) -> (165.5211, 24.3753)
  line L138 (165.9875, 28.7102) -> (166.0127, 25.2461)
  line L139 (162.0254, 23.4826) -> (165.0127, 25.2364)
  line L140 (169.5588, 19.2108) -> (172.5714, 17.5007)
  line L141 (165.5211, 24.3753) -> (162.5338, 22.6214)
  line L142 (166.0127, 25.2461) -> (169.0252, 23.536)
  line L143 (169.0252, 23.536) -> (172.0125, 25.2898)
  line L144 (165.0127, 25.2364) -> (164.9875, 28.7005)
  line L145 (161.975, 30.4106) -> (158.9877, 28.6567)
  line L146 (162.559, 19.1574) -> (165.5716, 17.4473)
  line L147 (172.0125, 25.2898) -> (171.9873, 28.7539)
  line L148 (175.5587, 19.2545) -> (175.5335, 22.7186)
  line L149 (175.5335, 22.7186) -> (172.5209, 24.4287)
  line L150 (182.5589, 19.2011) -> (182.5337, 22.6652)
  line L151 (185.9873, 28.7539) -> (182.9748, 30.464)
  line L152 (176.5338, 22.6214) -> (176.559, 19.1574)
  line L153 (173.0129, 25.1927) -> (176.0254, 23.4826)
  line L154 (182.9748, 30.464) -> (179.9875, 28.7102)
  line L155 (172.9877, 28.6567) -> (173.0129, 25.1927)
  line L156 (186.5714, 17.5007) -> (189.5587, 19.2545)
  line L157 (183.5336, 22.6749) -> (183.5588, 19.2108)
  line L158 (186.5209, 24.4287) -> (183.5336, 22.6749)
  line L159 (178.9875, 28.7005) -> (175.975, 30.4106)
  line L160 (179.5716, 17.4473) -> (182.5589, 19.2011)
  line L161 (182.5337, 22.6652) -> (179.5211, 24.3753)
  line L162 (179.9875, 28.7102) -> (180.0127, 25.2461)
  line L163 (176.0254, 23.4826) -> (179.0127, 25.2364)
  line L164 (183.5588, 19.2108) -> (186.5714, 17.5007)
  line L165 (179.5211, 24.3753) -> (176.5338, 22.6214)
  line L166 (180.0127, 25.2461) -> (183.0252, 23.536)
  line L167 (183.0252, 23.536) -> (186.0125, 25.2898)
  line L168 (179.0127, 25.2364) -> (178.9875, 28.7005)
  line L169 (175.975, 30.4106) -> (172.9877, 28.6567)
  line L170 (176.559, 19.1574) -> (179.5716, 17.4473)
  line L171 (186.0125, 25.2898) -> (185.9873, 28.7539)
  line L172 (189.5587, 19.2545) -> (189.5335, 22.7186)
  line L173 (189.5335, 22.7186) -> (186.5209, 24.4287)
  line L174 (196.5589, 19.2011) -> (196.5337, 22.6652)
  line L175 (199.9873, 28.7539) -> (196.9748, 30.464)
  line L176 (190.5338, 22.6214) -> (190.559, 19.1574)
  line L177 (187.0129, 25.1927) -> (190.0254, 23.4826)
  line L178 (196.9748, 30.464) -> (193.9875, 28.7102)
  line L179 (186.9877, 28.6567) -> (187.0129, 25.1927)
  line L180 (200.5714, 17.5007) -> (203.5587, 19.2545)
  line L181 (197.5336, 22.6749) -> (197.5588, 19.2108)
  line L182 (200.5209, 24.4287) -> (197.5336, 22.6749)
  line L183 (192.9875, 28.7005) -> (189.975, 30.4106)
  line L184 (193.5716, 17.4473) -> (196.5589, 19.2011)
  line L185 (196.5337, 22.6652) -> (193.5211, 24.3753)
  line L186 (193.9875, 28.7102) -> (194.0127, 25.2461)
  line L187 (190.0254, 23.4826) -> (193.0127, 25.2364)
  line L188 (197.5588, 19.2108) -> (200.5714, 17.5007)
  line L189 (193.5211, 24.3753) -> (190.5338, 22.6214)
  line L190 (194.0127, 25.2461) -> (197.0252, 23.536)
  line L191 (197.0252, 23.536) -> (200.0125, 25.2898)
  line L192 (193.0127, 25.2364) -> (192.9875, 28.7005)
  line L193 (189.975, 30.4106) -> (186.9877, 28.6567)
  line L194 (190.559, 19.1574) -> (193.5716, 17.4473)
  line L195 (200.0125, 25.2898) -> (199.9873, 28.7539)
  line L196 (203.5587, 19.2545) -> (203.5335, 22.7186)
  line L197 (203.5335, 22.7186) -> (200.5209, 24.4287)
  line L198 (210.5589, 19.2011) -> (210.5337, 22.6652)
  line L199 (213.9873, 28.7539) -> (210.9748, 30.464)
  line L200 (204.5338, 22.6214) -> (204.559, 19.1574)
  line L201 (201.0129, 25.1927) -> (204.0254, 23.4826)
  line L202 (210.9748, 30.464) -> (207.9875, 28.7102)
  line L203 (200.9877, 28.6567) -> (201.0129, 25.1927)
  line L204 (214.5714, 17.5007) -> (217.5587, 19.2545)
  line L205 (211.5336, 22.6749) -> (211.5588, 19.2108)
  line L206 (214.5209, 24.4287) -> (211.5336, 22.6749)
  line L207 (206.9875, 28.7005) -> (203.975, 30.4106)
  line L208 (207.5716, 17.4473) -> (210.5589, 19.2011)
  line L209 (210.5337, 22.6652) -> (207.5211, 24.3753)
  line L210 (207.9875, 28.7102) -> (208.0127, 25.2461)
  line L211 (204.0254, 23.4826) -> (207.0127, 25.2364)
  line L212 (211.5588, 19.2108) -> (214.5714, 17.5007)
  line L213 (207.5211, 24.3753) -> (204.5338, 22.6214)
  line L214 (208.0127, 25.2461) -> (211.0252, 23.536)
  line L215 (211.0252, 23.536) -> (214.0125, 25.2898)
  line L216 (207.0127, 25.2364) -> (206.9875, 28.7005)
  line L217 (203.975, 30.4106) -> (200.9877, 28.6567)
  line L218 (204.559, 19.1574) -> (207.5716, 17.4473)
  line L219 (214.0125, 25.2898) -> (213.9873, 28.7539)
  line L220 (217.5587, 19.2545) -> (217.5335, 22.7186)
  line L221 (217.5335, 22.7186) -> (214.5209, 24.4287)
  line L222 (224.5589, 19.2011) -> (224.5337, 22.6652)
  line L223 (227.9873, 28.7539) -> (224.9748, 30.464)
  line L224 (218.5338, 22.6214) -> (218.559, 19.1574)
  line L225 (215.0129, 25.1927) -> (218.0254, 23.4826)
  line L226 (224.9748, 30.464) -> (221.9875, 28.7102)
  line L227 (214.9877, 28.6567) -> (215.0129, 25.1927)
  line L228 (228.5714, 17.5007) -> (231.5587, 19.2545)
  line L229 (225.5336, 22.6749) -> (225.5588, 19.2108)
  line L230 (228.5209, 24.4287) -> (225.5336, 22.6749)
  line L231 (220.9875, 28.7005) -> (217.975, 30.4106)
  line L232 (221.5716, 17.4473) -> (224.5589, 19.2011)
  line L233 (224.5337, 22.6652) -> (221.5211, 24.3753)
  line L234 (221.9875, 28.7102) -> (222.0127, 25.2461)
  line L235 (218.0254, 23.4826) -> (221.0127, 25.2364)
  line L236 (225.5588, 19.2108) -> (228.5714, 17.5007)
  line L237 (221.5211, 24.3753) -> (218.5338, 22.6214)
  line L238 (222.0127, 25.2461) -> (225.0252, 23.536)
  line L239 (225.0252, 23.536) -> (228.0125, 25.2898)
  line L240 (221.0127, 25.2364) -> (220.9875, 28.7005)
  line L241 (217.975, 30.4106) -> (214.9877, 28.6567)
  line L242 (218.559, 19.1574) -> (221.5716, 17.4473)
  line L243 (228.0125, 25.2898) -> (227.9873, 28.7539)
  line L244 (231.5587, 19.2545) -> (231.5335, 22.7186)
  line L245 (231.5335, 22.7186) -> (228.5209, 24.4287)
  line L246 (140.5589, 31.2011) -> (140.5337, 34.6652)
  line L247 (143.9873, 40.7539) -> (140.9748, 42.464)
  line L248 (134.5338, 34.6214) -> (134.559, 31.1574)
  line L249 (131.0129, 37.1927) -> (134.0254, 35.4826)
  line L250 (140.9748, 42.464) -> (137.9875, 40.7102)
  line L251 (130.9877, 40.6567) -> (131.0129, 37.1927)
  line L252 (144.5714, 29.5007) -> (147.5587, 31.2545)
  line L253 (141.5336, 34.6749) -> (141.5588, 31.2108)
  line L254 (144.5209, 36.4287) -> (141.5336, 34.6749)
  line L255 (136.9875, 40.7005) -> (133.975, 42.4106)
  line L256 (137.5716, 29.4473) -> (140.5589, 31.2011)
  line L257 (140.5337, 34.6652) -> (137.5211, 36.3753)
  line L258 (137.9875, 40.7102) -> (138.0127, 37.2461)
  line L259 (134.0254, 35.4826) -> (137.0127, 37.2364)
  line L260 (141.5588, 31.2108) -> (144.5714, 29.5007)
  line L261 (137.5211, 36.3753) -> (134.5338, 34.6214)
  line L262 (138.0127, 37.2461) -> (141.0252, 35.536)
  line L263 (141.0252, 35.536) -> (144.0125, 37.2898)
  line L264 (137.0127, 37.2364) -> (136.9875, 40.7005)
  line L265 (133.975, 42.4106) -> (130.9877, 40.6567)
  line L266 (134.559, 31.1574) -> (137.5716, 29.4473)
  line L267 (144.0125, 37.2898) -> (143.9873, 40.7539)
  line L268 (147.5587, 31.2545) -> (147.5335, 34.7186)
  line L269 (147.5335, 34.7186) -> (144.5209, 36.4287)
  line L270 (154.5589, 31.2011) -> (154.5337, 34.6652)
  line L271 (157.9873, 40.7539) -> (154.9748, 42.464)
  line L272 (148.5338, 34.6214) -> (148.559, 31.1574)
  line L273 (145.0129, 37.1927) -> (148.0254, 35.4826)
  line L274 (154.9748, 42.464) -> (151.9875, 40.7102)
  line L275 (144.9877, 40.6567) -> (145.0129, 37.1927)
  line L276 (158.5714, 29.5007) -> (161.5587, 31.2545)
  line L277 (155.5336, 34.6749) -> (155.5588, 31.2108)
  line L278 (158.5209, 36.4287) -> (155.5336, 34.6749)
  line L279 (150.9875, 40.7005) -> (147.975, 42.4106)
  line L280 (151.5716, 29.4473) -> (154.5589, 31.2011)
  line L281 (154.5337, 34.6652) -> (151.5211, 36.3753)
  line L282 (151.9875, 40.7102) -> (152.0127, 37.2461)
  line L283 (148.0254, 35.4826) -> (151.0127, 37.2364)
  line L284 (155.5588, 31.2108) -> (158.5714, 29.5007)
  line L285 (151.5211, 36.3753) -> (148.5338, 34.6214)
  line L286 (152.0127, 37.2461) -> (155.0252, 35.536)
  line L287 (155.0252, 35.536) -> (158.0125, 37.2898)
  line L288 (151.0127, 37.2364) -> (150.9875, 40.7005)
  line L289 (147.975, 42.4106) -> (144.9877, 40.6567)
  line L290 (148.559, 31.1574) -> (151.5716, 29.4473)
  line L291 (158.0125, 37.2898) -> (157.9873, 40.7539)
  line L292 (161.5587, 31.2545) -> (161.5335, 34.7186)
  line L293 (161.5335, 34.7186) -> (158.5209, 36.4287)
  line L294 (168.5589, 31.2011) -> (168.5337, 34.6652)
  line L295 (171.9873, 40.7539) -> (168.9748, 42.464)
  line L296 (162.5338, 34.6214) -> (162.559, 31.1574)
  line L297 (159.0129, 37.1927) -> (162.0254, 35.4826)
  line L298 (168.9748, 42.464) -> (165.9875, 40.7102)
  line L299 (158.9877, 40.6567) -> (159.0129, 37.1927)
  line L300 (172.5714, 29.5007) -> (175.5587, 31.2545)
  line L301 (169.5336, 34.6749) -> (169.5588, 31.2108)
  line L302 (172.5209, 36.4287) -> (169.5336, 34.6749)
  line L303 (164.9875, 40.7005) -> (161.975, 42.4106)
  line L304 (165.5716, 29.4473) -> (168.5589, 31.2011)
  line L305 (168.5337, 34.6652) -> (165.5211, 36.3753)
  line L306 (165.9875, 40.7102) -> (166.0127, 37.2461)
  line L307 (162.0254, 35.4826) -> (165.0127, 37.2364)
  line L308 (169.5588, 31.2108) -> (172.5714, 29.5007)
  line L309 (165.5211, 36.3753) -> (162.5338, 34.6214)
  line L310 (166.0127, 37.2461) -> (169.0252, 35.536)
  line L311 (169.0252, 35.536) -> (172.0125, 37.2898)
  line L312 (165.0127, 37.2364) -> (164.9875, 40.7005)
  line L313 (161.975, 42.4106) -> (158.9877, 40.6567)
  line L314 (162.559, 31.1574) -> (165.5716, 29.4473)
  line L315 (172.0125, 37.2898) -> (171.9873, 40.7539)
  line L316 (175.5587, 31.2545) -> (175.5335, 34.7186)
  line L317 (175.5335, 34.7186) -> (172.5209, 36.4287)
  line L318 (182.5589, 31.2011) -> (182.5337, 34.6652)
  line L319 (185.9873, 40.7539) -> (182.9748, 42.464)
  line L320 (176.5338, 34.6214) -> (176.559, 31.1574)
  line L321 (173.0129, 37.1927) -> (176.0254, 35.4826)
  line L322 (182.9748, 42.464) -> (179.9875, 40.7102)
  line L323 (172.9877, 40.6567) -> (173.0129, 37.1927)
  line L324 (186.5714, 29.5007) -> (189.5587, 31.2545)
  line L325 (183.5336, 34.6749) -> (183.5588, 31.2108)
  line L326 (186.5209, 36.4287) -> (183.5336, 34.6749)
  line L327 (178.9875, 40.7005) -> (175.975, 42.4106)
  line L328 (179.5716, 29.4473) -> (182.5589, 31.2011)
  line L329 (182.5337, 34.6652) -> (179.5211, 36.3753)
  line L330 (179.9875, 40.7102) -> (180.0127, 37.2461)
  line L331 (176.0254, 35.4826) -> (179.0127, 37.2364)
  line L332 (183.5588, 31.2108) -> (186.5714, 29.5007)
  line L333 (179.5211, 36.3753) -> (176.5338, 34.6214)
  line L334 (180.0127, 37.2461) -> (183.0252, 35.536)
  line L335 (183.0252, 35.536) -> (186.0125, 37.2898)
  line L336 (179.0127, 37.2364) -> (178.9875, 40.7005)
  line L337 (175.975, 42.4106) -> (172.9877, 40.6567)
  line L338 (176.559, 31.1574) -> (179.5716, 29.4473)
  line L339 (186.0125, 37.2898) -> (185.9873, 40.7539)
  line L340 (189.5587, 31.2545) -> (189.5335, 34.7186)
  line L341 (189.5335, 34.7186) -> (186.5209, 36.4287)
  line L342 (196.5589, 31.2011) -> (196.5337, 34.6652)
  line L343 (199.9873, 40.7539) -> (196.9748, 42.464)
  line L344 (190.5338, 34.6214) -> (190.559, 31.1574)
  line L345 (187.0129, 37.1927) -> (190.0254, 35.4826)
  line L346 (196.9748, 42.464) -> (193.9875, 40.7102)
  line L347 (186.9877, 40.6567) -> (187.0129, 37.1927)
  line L348 (200.5714, 29.5007) -> (203.5587, 31.2545)
  line L349 (197.5336, 34.6749) -> (197.5588, 31.2108)
  line L350 (200.5209, 36.4287) -> (197.5336, 34.6749)
  line L351 (192.9875, 40.7005) -> (189.975, 42.4106)
  line L352 (193.5716, 29.4473) -> (196.5589, 31.2011)
  line L353 (196.5337, 34.6652) -> (193.5211, 36.3753)
  line L354 (193.9875, 40.7102) -> (194.0127, 37.2461)
  line L355 (190.0254, 35.4826) -> (193.0127, 37.2364)
  line L356 (197.5588, 31.2108) -> (200.5714, 29.5007)
  line L357 (193.5211, 36.3753) -> (190.5338, 34.6214)
  line L358 (194.0127, 37.2461) -> (197.0252, 35.536)
  line L359 (197.0252, 35.536) -> (200.0125, 37.2898)
  line L360 (193.0127, 37.2364) -> (192.9875, 40.7005)
  line L361 (189.975, 42.4106) -> (186.9877, 40.6567)
  line L362 (190.559, 31.1574) -> (193.5716, 29.4473)
  line L363 (200.0125, 37.2898) -> (199.9873, 40.7539)
  line L364 (203.5587, 31.2545) -> (203.5335, 34.7186)
  line L365 (203.5335, 34.7186) -> (200.5209, 36.4287)